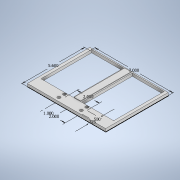
# Autodesk Inventor part: USAXS double well plate
Saved by Autodesk Inventor 2020 (Build 240168000, 168)
## iProperties
Created: 2022-06-26
Part Number: USAXS double well plate
Material: Generic
Document SubType Name: Modeling
Designer: Beaucage
Density: 1 g/cm^3
Appearance: Default
Author: Beaucage
Autodesk Inventor part; units mm, degrees
ref_plane "YZ Plane" through (0, 0, 0) normal (1, 0, 0) x (0, 1, 0)
ref_plane "XZ Plane" through (0, 0, 0) normal (0, 1, 0) x (-1, 0, 0)
ref_plane "XY Plane" through (0, 0, 0) normal (0, 0, 1) x (1, 0, 0)
sketch "Sketch1" plane through (0, 0, 0) normal (0, 1, 0) x (-1, 0, 0)
  line L0 (0, 0) -> (177.8, 0)
  line L1 (177.8, 0) -> (177.8, -142.24)
  line L2 (177.8, -142.24) -> (0, -142.24)
  line L3 (0, -142.24) -> (0, 0)
  line L4 (177.8, 0) -> (88.9, 0)
  line L5 (88.9, 0) -> (114.3, 0)
  line L6 (114.3, 0) -> (63.5, 0)
  line L7 (63.5, 0) -> (63.5, -8.255)
  line L8 (63.5, -8.255) -> (63.5, -20.955)
  line L9 (63.5, -20.955) -> (114.3, -20.955)
  line L10 (114.3, -20.955) -> (114.3, -8.255)
  point P0 (116.227, -12.0777)
  dimension "d0" = 177.8
  dimension "d1" = 142.24
  dimension "d2" = 25.4
  dimension "d3" = 50.8
  dimension "d4" = 8.255
  dimension "d5" = 12.7
  dimension "d6" = 50.8
  constraints: 22 end point, 4 perpendicular, 3 point on line, 2 parallel, 1 horizontal, 1 midpoint
  measures "d0" distance of L1.end L2.end
  measures "d1" distance of L0.end L1.end
  measures "d2" distance of L4.end L5.end
  measures "d3" distance of L5.end L6.end
  measures "d4" distance of L6.end L7.end
  measures "d5" distance of L7.end L8.end
  measures "d6" distance of L8.end L9.end
extrude "Extrusion1" add sketch "Sketch1" along normal blind 6.35
hole "Hole1" at (-63.5, 0, -8.255) at (-63.5, 0, -20.955) at (-114.3, 0, -20.955) at (-114.3, 0, -8.255) direction (0, 1, 0) diameter 6.7564 end through all clearance for "Socket Head Cap Screw" size "1/4" standard "Ansi Unified Screw Threads"
sketch "Sketch2" plane through (0, 6.35, 0) normal (0, 1, 0) x (1, 0, 0)
  line L0 (-177.8, 142.24) -> (-177.8, 0) projected
  line L1 (-177.8, 142.24) -> (-171.45, 142.24)
  line L2 (-171.45, 142.24) -> (-171.45, 139.7)
  line L3 (-171.45, 139.7) -> (-177.8, 139.7)
  line L4 (-177.8, 139.7) -> (-177.8, 142.24)
  line L5 (-171.45, 139.7) -> (-98.6688, 139.7)
  line L6 (-98.6688, 139.7) -> (-98.6688, 24.6405)
  line L7 (-98.6688, 24.6405) -> (-171.45, 24.6405)
  line L8 (-171.45, 24.6405) -> (-171.45, 139.7)
  line L9 (0, 142.24) -> (-177.8, 142.24) projected
  line L10 (0, 142.24) -> (-6.35, 142.24)
  line L11 (-6.35, 142.24) -> (-6.35, 139.7)
  line L12 (-6.35, 139.7) -> (0, 139.7)
  line L13 (0, 139.7) -> (0, 142.24)
  line L14 (-6.35, 139.7) -> (-79.121, 139.7)
  line L15 (-79.121, 139.7) -> (-79.121, 24.6405)
  line L16 (-79.121, 24.6405) -> (-6.35, 24.6405)
  line L17 (-6.35, 24.6405) -> (-6.35, 139.7)
  point P0 (0, 0)
  dimension "d16" = 6.35
  dimension "d17" = 2.54
  dimension "d18" = 72.7812
  dimension "d19" = 115.0595
  dimension "d20" = 6.35
  dimension "d21" = 72.771
  dimension "d22" = 115.0595
  constraints: 32 end point, 8 parallel, 4 horizontal, 4 perpendicular
  measures "d16" distance of L2.end L3.end
  measures "d17" distance of L1.end L2.end
  measures "d18" distance of L6.end L7.end
  measures "d19" distance of L5.end L6.end
  measures "d20" distance of L12.end L11.end
  measures "d21" distance of L16.end L15.end
  measures "d22" distance of L15.end L14.end
extrude "Extrusion2" cut sketch "Sketch2" against normal blind 6.35 contours L17 L16 L15 L14 | L5 L6 L7 L8
sketch "Sketch3" plane through (0, 6.35, 0) normal (0, 1, 0) x (1, 0, 0)
  line L0 (-98.6688, 139.7) -> (-171.45, 139.7) projected
  line L1 (-98.6688, 139.7) -> (-96.1288, 139.7)
  line L2 (-96.1288, 139.7) -> (-96.1288, 24.6405)
  line L3 (-96.1288, 24.6405) -> (-98.6688, 24.6405)
  line L4 (-98.6688, 24.6405) -> (-98.6688, 139.7)
  line L5 (-79.121, 24.6405) -> (-79.121, 139.7) projected
  line L6 (-79.121, 24.6405) -> (-81.661, 24.6405)
  line L7 (-81.661, 24.6405) -> (-81.661, 139.7)
  line L8 (-81.661, 139.7) -> (-79.121, 139.7)
  line L9 (-79.121, 139.7) -> (-79.121, 24.6405)
  line L10 (-96.1288, 139.7) -> (-93.5888, 139.7)
  line L11 (-93.5888, 139.7) -> (-93.5888, 24.6405)
  line L12 (-93.5888, 24.6405) -> (-96.1288, 24.6405)
  line L13 (-96.1288, 24.6405) -> (-96.1288, 139.7)
  line L14 (-81.661, 24.6405) -> (-84.201, 24.6405)
  line L15 (-84.201, 24.6405) -> (-84.201, 139.7)
  line L16 (-84.201, 139.7) -> (-81.661, 139.7)
  line L17 (-81.661, 139.7) -> (-81.661, 24.6405)
  line L18 (-93.5888, 139.7) -> (-84.201, 139.7)
  line L19 (-84.201, 139.7) -> (-84.201, 24.6405)
  line L20 (-84.201, 24.6405) -> (-93.5888, 24.6405)
  line L21 (-93.5888, 24.6405) -> (-93.5888, 139.7)
  point P0 (0, 0)
  dimension "d26" = 2.54
  dimension "d27" = 2.54
  dimension "d30" = 2.54
  dimension "d31" = 2.54
  constraints: 40 end point, 10 parallel, 5 horizontal, 5 perpendicular, 2 point on line
  measures "d26" distance of L2.end L3.end
  measures "d27" distance of L7.end L8.end
  measures "d30" distance of L11.end L12.end
  measures "d31" distance of L15.end L16.end
extrude "Extrusion4" add sketch "Sketch3" along normal blind 1.27 contours L10 L11 L12 L2 | L18 L15 L20 L11 | L16 L7 L14 L15
body "Solid1"
